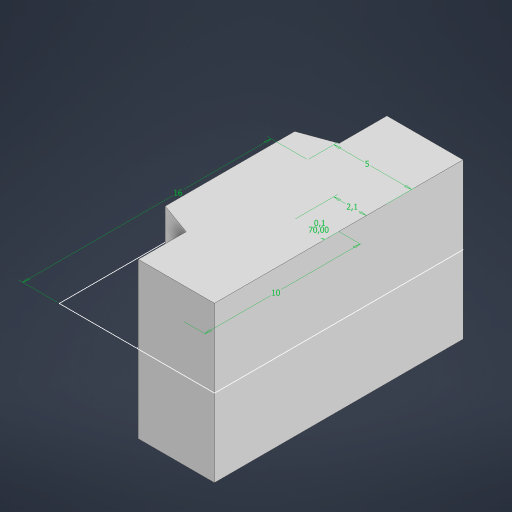
# Autodesk Inventor part: bat_contacts_v2_contact_form1
Saved by Autodesk Inventor 2024.3 (Build 283343010, 343A)
## iProperties
Created: 2025-05-21
Part Number: bat_contacts_v2_contact_form1
Material: Generisch
Document SubType Name: Modeling
Designer: David
Density: 1 g/cm^3
Appearance: Vorgabe
Author: David
## iProperties of the stored document bat_contacts_v2_contact_form1_3D-Druck.ipt
Created: 2025-05-21
Part Number: bat_contacts_v2_contact_form1_3D-Druck
Material: Generisch
Document SubType Name: Modeling
Designer: David
Density: 1 g/cm^3
Appearance: Vorgabe
Author: David
Autodesk Inventor part; units mm, degrees
ref_plane "YZ Plane" through (0, 0, 0) normal (1, 0, 0) x (0, 1, 0)
ref_plane "XZ Plane" through (0, 0, 0) normal (0, 1, 0) x (-1, 0, 0)
ref_plane "XY Plane" through (0, 0, 0) normal (0, 0, 1) x (1, 0, 0)
sketch "Skizze1" plane through (0, 0, 0) normal (0, 0, 1) x (1, 0, 0)
  line L0 (0, 3) -> (0, 0)
  line L1 (0, 0) -> (-2.1, -0.7643)
  line L2 (-2.1, -0.7643) -> (-2.1, -9.2357)
  line L3 (-2.1, -9.2357) -> (0, -10)
  line L4 (0, -10) -> (0, -13)
  line L5 (0, 3) -> (-5, 3)
  line L6 (-5, 3) -> (-5, -13)
  line L7 (-5, -13) -> (0, -13)
  line L8 (0, 3) -> (5, 3)
  line L9 (5, 3) -> (5, -13)
  line L10 (5, -13) -> (0, -13)
  line L11 (0.1, -13) -> (0.1, -9.93)
  line L12 (0.1, -9.93) -> (-2, -9.1656)
  line L13 (-2, -9.1656) -> (-2, -0.8344)
  line L14 (-2, -0.8344) -> (0.1, -0.07)
  line L15 (0.1, -0.07) -> (0.1, 3)
  line L16 (0, 0) -> (0, -10)
  point P0 (0, -9.8936)
  point P1 (0, -0.1064)
  dimension "d0" = 2.1
  dimension "d1" = 10
  dimension "d2" = 70
  dimension "d3" = 5
  dimension "d4" = 16
  dimension "d5" = 0.1
  constraints: 34 end point, 4 point on line, 3 equal length, 3 horizontal, 3 perpendicular, 2 parallel, 2 vertical, 4 other
  measures "d0" distance between parallel lines of L0 L2
  measures "d1" distance of L3.end L0.end
  measures "d2" angle of L0 L1
  measures "d3" distance of L0.start L5.end
  measures "d4" distance of L5.end L6.end
  measures "d5" distance between parallel lines of L1 L14
extrude "Extrusion3" add sketch "Skizze1" along normal mid plane 10 contours L8 L9 L10 L11 L12 L16 L14 L15 | L16 L12 L13 L14
